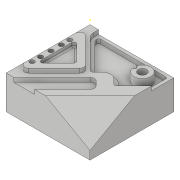
# Autodesk Inventor part: proyecto
Saved by Autodesk Inventor 2018 (Build 220112000, 112)
## iProperties
Created: 2018-04-26
Part Number: proyecto
Material: Generic
Document SubType Name: Modeling
Designer: SONY
Density: 1 g/cm^3
Appearance: Default
Author: SONY
Autodesk Inventor part; units mm, degrees
ref_plane "YZ Plane" through (0, 0, 0) normal (1, 0, 0) x (0, 1, 0)
ref_plane "XZ Plane" through (0, 0, 0) normal (0, 1, 0) x (-1, 0, 0)
sketch "Sketch1" plane through (0, 0, 0) normal (0, 0, 1) x (1, 0, 0)
  line L0 (0, 0) -> (200, 0)
  line L1 (200, 0) -> (200, 80)
  line L2 (200, 80) -> (0, 80)
  line L3 (0, 80) -> (0, 0)
  dimension "d0" = 200
  dimension "d1" = 80
  constraints: 8 end point, 2 parallel, 1 horizontal, 1 perpendicular
  measures "d0" distance of L2.end L1.end
  measures "d1" distance of L0.end L1.end
extrude "Extrusion1" add sketch "Sketch1" along normal blind 200
sketch "Sketch2" plane through (0, 80, 0) normal (0, 1, 0) x (1, 0, 0)
  line L0 (0, 0) -> (200, 0) projected
  line L1 (0, 0) -> (0, -200) projected
  line L2 (10, -20.6066) -> (10, -190)
  line L3 (20.6066, -10) -> (190, -10)
  line L4 (10, -20.6066) -> (10, -25)
  line L5 (20.6066, -10) -> (25, -10)
  line L6 (105.3033, -94.6967) -> (20.6066, -10)
  line L7 (94.6967, -105.3033) -> (10, -20.6066)
  line L8 (190, -10) -> (105.3033, -94.6967)
  line L9 (94.6967, -105.3033) -> (10, -190)
  line L10 (105.3033, -73.4835) -> (153.7868, -25)
  line L11 (94.6967, -105.3033) -> (84.0901, -115.9099)
  line L12 (73.4835, -105.3033) -> (25, -56.8198)
  line L13 (105.3033, -73.4835) -> (56.8198, -25)
  line L14 (153.7868, -25) -> (56.8198, -25)
  line L15 (25, -56.8198) -> (25, -153.7868)
  line L16 (134.3503, -134.3503) -> (91.9239, -176.7767)
  line L17 (63.6396, -148.4924) -> (148.4924, -63.6396)
  line L18 (176.7767, -91.9239) -> (134.3503, -134.3503)
  arc A0 (176.7767, -91.9239) -> (148.4924, -63.6396) centre (162.6346, -77.7817) ccw
  arc A1 (169.7056, -84.8528) -> (155.5635, -70.7107) centre (162.6346, -77.7817) ccw
  line L19 (169.7056, -84.8528) -> (97.1003, -157.4582)
  line L20 (155.5635, -70.7107) -> (82.9581, -143.316)
  line L21 (73.4835, -105.3033) -> (25, -153.7868)
  line L22 (10, -110.6066) -> (25, -110.6066)
  circle A2 centre (17.5, -110.6066) radius 5.5
  circle A3 centre (17.5, -135.6066) radius 5.5
  circle A4 centre (17.5, -85.6066) radius 5.5
  circle A5 centre (17.5, -65.6066) radius 3.5
  circle A6 centre (17.5, -155.6066) radius 3.5
  arc A7 (63.6396, -148.4924) -> (91.9239, -176.7767) centre (77.7817, -162.6346) ccw
  arc A8 (97.1003, -157.4582) -> (82.9581, -143.316) centre (77.7817, -162.6346) ccw
  dimension "d20" = 40
  dimension "d22" = 11
  dimension "d24" = 11
  dimension "d26" = 11
  dimension "d29" = 7
  dimension "d30" = 7
  constraints: 42 end point, 9 centre point, 8 point on circle, 6 point on line, 2 parallel, 2 tangent, 1 coincident, 1 horizontal, 1 perpendicular, 1 vertical
  measures "d20" distance of L16.end L17.start
  measures "d22" diameter of A2
  measures "d24" diameter of A3
  measures "d26" diameter of A4
  measures "d29" diameter of A5
  measures "d30" diameter of A6
extrude "Extrusion2" add sketch "Sketch2" along normal blind 10
ref_plane "Work Plane1" through (0, 80, 0) normal (-0.7071, 0, 0.7071) x (0, -1, 0)
sketch "Sketch3" plane through (0, 80, 0) normal (-0.7071, 0, 0.7071) x (0, -1, 0)
  line L0 (80, 282.8427) -> (0, 282.8427) projected
  line L1 (0, 282.8427) -> (0, 207.8427)
  line L2 (0, 141.4214) -> (0, 282.8427) projected
  line L3 (0, 282.8427) -> (60, 282.8427)
  line L4 (60, 282.8427) -> (0, 207.8427)
  point P0 (80, 0)
  dimension "d33" = 75
  dimension "d34" = 60
  constraints: 6 end point, 1 point on line, 1 vertical
  measures "d33" distance of L0.end L1.end
  measures "d34" distance of L0.end L3.end
extrude "Extrusion3" cut sketch "Sketch3" along normal mid plane 200
fillet "Fillet1" radius 5 3 edges at (25, 85, 56.8198) (73.4835, 85, 105.3033) (25, 85, 153.7868)
sketch "Sketch5" plane through (0, 90, 0) normal (0, 1, 0) x (1, 0, 0)
  point P0 (0, 0)
sketch "Sketch6" plane through (0, 90, 0) normal (0, 1, 0) x (1, 0, 0)
  arc A0 (63.6396, -148.4924) -> (91.9239, -176.7767) centre (77.7817, -162.6346) ccw projected
  arc A1 (63.6396, -148.4924) -> (91.9239, -176.7767) centre (77.7817, -162.6346) ccw
  arc A2 (169.7056, -84.8528) -> (155.5635, -70.7107) centre (162.6346, -77.7817) ccw projected
  arc A3 (176.7767, -91.9239) -> (148.4924, -63.6396) centre (162.6346, -77.7817) ccw
  line L0 (148.4924, -63.6396) -> (63.6396, -148.4924) projected
  line L1 (63.6396, -148.4924) -> (148.4924, -63.6396)
  line L2 (91.9239, -176.7767) -> (176.7767, -91.9239) projected
  line L3 (91.9239, -176.7767) -> (176.7767, -91.9239)
  point P0 (0, 0)
  constraints: 5 end point, 4 point on circle, 2 centre point, 2 coincident, 2 collinear, 1 tangent
extrude "Extrusion5" cut sketch "Sketch6" against normal blind 10
sketch "Sketch7" plane through (0, 90, 0) normal (0, 1, 0) x (1, 0, 0)
  line L0 (105.3033, -94.6967) -> (20.6066, -10) projected
  line L1 (20.6066, -10) -> (105.3033, -94.6967)
  line L2 (190, -10) -> (105.3033, -94.6967) projected
  line L3 (105.3033, -94.6967) -> (190, -10)
  line L4 (190, -10) -> (20.6066, -10)
  point P0 (0, 0)
  constraints: 6 end point, 2 collinear, 1 horizontal
extrude "Extrusion6" cut sketch "Sketch7" against normal blind 10
sketch "Sketch8" plane through (0, 80, 0) normal (0, 1, 0) x (1, 0, 0)
  line L0 (200, 0) -> (0, 0) projected
  line L1 (0, 0) -> (20.645, 0)
  line L2 (20.645, 0) -> (20.645, -20)
  line L3 (20.645, -20) -> (126.7111, -126.066)
  line L4 (20.645, -20) -> (170.645, -20) construction
  line L5 (126.7111, -126.066) -> (200, -52.7771)
  line L6 (200, 0) -> (200, -93.934) projected
  line L7 (20.645, 0) -> (200, 0)
  line L8 (200, -52.7771) -> (200, 0)
  dimension "d45" = 20
  dimension "d46" = 150
  dimension "d47" = 45
  constraints: 14 end point, 3 perpendicular, 2 point on line, 1 equal length, 1 horizontal, 1 parallel
  measures "d45" distance of L1.end L2.end
  measures "d46" distance of L2.end L3.end
  measures "d47" angle of L3 L4
extrude "Extrusion7" cut sketch "Sketch8" against normal blind 10
fillet "Fillet2" radius 20 2 edges at (126.7111, 75, 126.066) (20.645, 75, 20)
sketch "Sketch9" plane through (0, 70, 0) normal (0, 1, 0) x (1, 0, 0)
  arc A0 (112.5689, -111.9239) -> (140.8532, -111.9239) centre (126.7111, -97.7817) ccw projected
  arc A1 (117.4902, -106.2213) -> (135.9319, -106.2213) centre (126.7111, -97.7817) ccw
  arc A2 (20.645, -11.7157) -> (26.5029, -25.8579) centre (40.645, -11.7157) ccw projected
  arc A3 (28.145, -11.7157) -> (31.8071, -20.5555) centre (40.645, -11.7157) ccw
  line L0 (117.4902, -106.2213) -> (31.8071, -20.5555)
  line L1 (135.9319, -106.2213) -> (226.547, -106.2213) construction
  line L2 (200, 0) -> (200, -52.7771) projected
  line L3 (200, 0) -> (192.5, 0)
  line L4 (20.645, 0) -> (200, 0) projected
  line L5 (192.5, -7.5) -> (192.5, -49.6532)
  line L6 (200, 0) -> (200, -7.5)
  line L7 (192.5, -7.5) -> (28.145, -7.5)
  line L8 (28.145, -11.7157) -> (28.145, -7.5)
  line L9 (135.9319, -106.2213) -> (192.5, -49.6532)
  line L10 (200, -42.1532) -> (200.0065, -42.1467)
  line L11 (126.7111, -97.7817) -> (126.7111, -85.2817)
  circle A4 centre (126.7111, -97.7817) radius 12.5
  point P0 (0, 0)
  dimension "d51" = 25
  dimension "d52" = 25
  dimension "d54" = 7.5
  dimension "d55" = 7.5
  constraints: 20 end point, 5 point on circle, 3 centre point, 3 coincident, 3 perpendicular, 3 point on line, 1 horizontal, 1 parallel, 1 tangent, 1 vertical
  measures "d51" diameter of A1
  measures "d52" diameter of A3
  measures "d54" distance of L2.start L3.end
  measures "d55" distance of L2.start L6.end
extrude "Extrusion8" cut sketch "Sketch9" against normal blind 10 contours L0 A3 L8 L7 L5 L9 A4
sketch "Sketch10" plane through (0, 70, 0) normal (0, 1, 0) x (1, 0, 0)
  arc A0 (135.9319, -106.2213) -> (117.4902, -106.2213) centre (126.7111, -97.7817) ccw projected
  circle A1 centre (126.7111, -97.7817) radius 20
  point P0 (0, 0)
  constraints: 1 centre point, 1 coincident
extrude "Extrusion9" add sketch "Sketch10" along normal blind 10 and the other way blind 10
sketch "Sketch11" plane through (0, 80, 200) normal (0, 1, 0) x (1, 0, 0)
  arc A0 (146.5879, 104.4347) -> (106.834, 104.4327) centre (126.7111, 102.2183) ccw projected
  line L0 (126.7111, 102.2183) -> (112.5689, 116.3604)
  line L1 (126.7111, 102.2183) -> (146.7111, 102.2183) construction
  line L2 (112.5689, 116.3604) -> (98.4268, 102.2183)
  line L3 (112.5689, 88.0761) -> (26.5029, 174.1421) projected
  line L4 (140.8532, 116.3604) -> (154.9953, 102.2183)
  line L5 (200, 147.2229) -> (140.8532, 88.0761) projected
  arc A1 (112.5689, 88.0761) -> (140.8532, 88.0761) centre (126.7111, 102.2183) ccw
  arc A2 (140.8532, 116.3604) -> (112.5689, 116.3604) centre (126.7111, 102.2183) ccw
  line L6 (112.5689, 88.0761) -> (98.4268, 102.2183)
  line L7 (154.9953, 102.2183) -> (140.8532, 88.0761)
  point P0 (0, 200)
  dimension "d62" = 135
  constraints: 14 end point, 4 point on circle, 2 centre point, 2 collinear, 2 perpendicular, 2 point on line, 1 coincident, 1 equal length, 1 horizontal, 1 tangent
  measures "d62" angle of L1 L0
extrude "Extrusion10" add sketch "Sketch11" against normal blind 20
fillet "Fillet3" radius 10 2 edges at (103.7373, 65, 92.4712) (149.6834, 65, 92.4698)
sketch "Sketch12" plane through (0, 70, 0) normal (0, 1, 0) x (1, 0, 0)
  arc A0 (140.8532, -83.6396) -> (112.5689, -83.6396) centre (126.7111, -97.7817) ccw projected
  line L0 (107.8365, -77.7817) -> (93.1316, -92.4866)
  line L1 (98.4268, -97.7817) -> (26.5029, -25.8579) projected
  line L2 (146.1565, -78.3363) -> (160.2986, -92.4784)
  line L3 (200, -52.7771) -> (154.9953, -97.7817) projected
  line L4 (160.2986, -92.4784) -> (127.5069, -125.2702)
  line L5 (127.5069, -125.2702) -> (93.9274, -91.6908)
  arc A1 (146.1565, -78.3363) -> (106.7111, -78.9072) centre (126.7111, -97.7817) ccw
  point P0 (0, 0)
  constraints: 8 end point, 4 point on line, 3 perpendicular, 3 point on circle, 1 centre point, 1 coincident, 1 tangent
extrude "Extrusion11" add sketch "Sketch12" against normal blind 20 contours A1 L2 L3 L4 L5 L0
fillet "Fillet4" radius 5 2 edges at (98.6681, 65, 86.9501) (154.7622, 65, 86.942)
fillet "Fillet5" radius 5 2 edges at (98.4268, 75, 97.7817) (154.9953, 75, 97.7817)
fillet "Fillet6" radius 5 3 edges at (192.5, 65, 7.5) (192.5, 65, 49.6532) (28.145, 65, 7.5)
sketch "Sketch13" plane through (0, 60, 0) normal (0, 1, 0) x (1, 0, 0)
  line L0 (200, 0) -> (200, -52.7771) projected
  line L1 (200, 0) -> (200, -35)
  line L2 (200, -35) -> (160, -35)
  circle A0 centre (160, -35) radius 20
  circle A1 centre (160, -35) radius 10
  point P0 (0, 0)
  dimension "d72" = 35
  dimension "d73" = 40
  dimension "d74" = 40
  dimension "d75" = 20
  constraints: 4 end point, 2 centre point, 2 coincident, 1 perpendicular, 1 point on line
  measures "d72" distance of L0.start L1.end
  measures "d73" distance of L1.end L2.end
  measures "d74" diameter of A0
  measures "d75" diameter of A1
extrude "Extrusion12" add sketch "Sketch13" along normal blind 20
fillet "Fillet7" radius 10 3 edges at (94.6967, 85, 105.3033) (10, 85, 20.6066) (10, 85, 190)
fillet "Fillet8" radius 3 6 edges at (28.0866, 80, 146.3351) (51.7417, 80, 127.045) (71.4124, 80, 105.3033) (51.7417, 80, 83.5616) (28.0866, 80, 64.2715) (25, 80, 105.3033)
sketch "Sketch14" plane through (160, 80, 35) normal (0, 1, 0) x (1, 0, 0)
  circle A0 centre (0, 0) radius 20 projected
  circle A1 centre (-20, 0) radius 5.5
  point P0 (-160, 35)
  dimension "d80" = 11
  constraints: 1 centre point, 1 horizontal alignment, 1 other
  measures "d80" diameter of A1
extrude "Extrusion13" cut sketch "Sketch14" against normal blind 20 contours A1 A0 | A0 A1 picked at (-18.1103, 0) picked at (-21.777, 0)
sketch "Sketch15" plane through (0, 80, 200) normal (0, 1, 0) x (1, 0, 0)
  line L0 (87.6256, 87.6256) -> (27.0711, 27.0711) projected
  line L1 (27.0711, 27.0711) -> (87.6256, 87.6256)
  line L2 (87.6256, 87.6256) -> (27.0711, 27.0711)
  line L3 (36.3259, 18.3055) -> (116.2946, 98.2741)
  line L4 (116.2946, 98.2741) -> (18.0204, 0)
  line L5 (116.2946, 98.2741) -> (141.0433, 73.5254)
  line L6 (141.0433, 73.5254) -> (67.5179, 0)
  line L7 (93.934, 0) -> (0, 0) projected
  line L8 (67.5179, 0) -> (18.0204, 0)
  point P0 (0, 200)
  dimension "d83" = 35
  constraints: 14 end point, 3 collinear, 2 point on line, 1 parallel, 1 perpendicular
  measures "d83" distance of L3.end L5.end
extrude "Extrusion14" cut sketch "Sketch15" against normal blind 10
fillet "Fillet9" radius 10 2 edges at (116.2946, 75, 101.7259) (141.0433, 75, 126.4746)
sketch "Sketch17" plane through (0, 90, 0) normal (0, 1, 0) x (1, 0, 0)
  circle A0 centre (17.5, -110.6066) radius 5.5 projected
  circle A1 centre (17.5, -110.6066) radius 5.5
  circle A2 centre (17.5, -135.6066) radius 5.5 projected
  circle A3 centre (17.5, -135.6066) radius 5.5
  circle A4 centre (17.5, -85.6066) radius 5.5 projected
  circle A5 centre (17.5, -85.6066) radius 5.5
  circle A6 centre (17.5, -65.6066) radius 3.5 projected
  circle A7 centre (17.5, -65.6066) radius 3.5
  circle A8 centre (17.5, -155.6066) radius 3.5 projected
  circle A9 centre (17.5, -155.6066) radius 3.5
  point P0 (0, 0)
  constraints: 5 centre point, 5 coincident
hole "Hole1" at (17.5, 90, 85.6066) at (17.5, 90, 110.6066) at (17.5, 90, 135.6066) direction (0, -1, 0) diameter 11 depth 25 tip angle 118
sketch "Sketch18" plane through (0, 90, 0) normal (0, 1, 0) x (1, 0, 0)
  circle A0 centre (17.5, -65.6066) radius 3.5 projected
  circle A1 centre (17.5, -65.6066) radius 3.5
  circle A2 centre (17.5, -155.6066) radius 3.5 projected
  circle A3 centre (17.5, -155.6066) radius 3.5
  point P0 (0, 0)
  constraints: 2 centre point, 2 coincident
hole "Hole2" at (17.5, 90, 65.6066) at (17.5, 90, 155.6066) direction (0, -1, 0) diameter 11 depth 25 tip angle 118
thread "Thread1" size "M11x1.5" class "6H" standard "ANSI Metric M Profile" length 15
thread "Thread2" size "M11x1.5" class "6H" standard "ANSI Metric M Profile" length 15
thread "Thread3" size "M11x1.5" class "6H" standard "ANSI Metric M Profile" length 15
body "Solid1"
